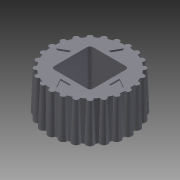
# Autodesk Inventor part: Shaft Lock Bar Insert
Saved by Autodesk Inventor 2013 (Build 170138000, 138)
## iProperties
Created: 2010-06-22
Part Number: Shaft Lock Bar Insert
Document SubType Name: Modeling
Designer: Phil
Density: 1 g/cm^3
Material: Generic
Author: Phil
Autodesk Inventor part; units mm, degrees
ref_plane "YZ Plane" through (0, 0, 0) normal (1, 0, 0) x (0, 1, 0)
ref_plane "XZ Plane" through (0, 0, 0) normal (0, 1, 0) x (-1, 0, 0)
ref_plane "XY Plane" through (0, 0, 0) normal (0, 0, 1) x (1, 0, 0)
sketch "Sketch1" plane through (0, 0, 0) normal (0, 0, 1) x (1, 0, 0)
  arc A0 (-3.0987, -0.2197) -> (-3.05, -0.5898) centre (0, 0) ccw projected
  arc A1 (-3.0987, 0.2197) -> (-3.0987, -0.2197) centre (-3.14, 0) ccw projected
  arc A2 (-3.05, 0.5898) -> (-3.0987, 0.2197) centre (0, 0) ccw projected
  arc A3 (-2.9362, 1.0142) -> (-3.05, 0.5898) centre (-3.033, 0.8127) ccw projected
  arc A4 (-2.7934, 1.3591) -> (-2.9362, 1.0142) centre (0, 0) ccw projected
  arc A5 (-2.5737, 1.7396) -> (-2.7934, 1.3591) centre (-2.7193, 1.57) ccw projected
  arc A6 (-2.3465, 2.0357) -> (-2.5737, 1.7396) centre (0, 0) ccw projected
  arc A7 (-2.0357, 2.3465) -> (-2.3465, 2.0357) centre (-2.2203, 2.2203) ccw projected
  arc A8 (-1.7396, 2.5737) -> (-2.0357, 2.3465) centre (0, 0) ccw projected
  arc A9 (-1.3591, 2.7934) -> (-1.7396, 2.5737) centre (-1.57, 2.7193) ccw projected
  arc A10 (-1.0142, 2.9362) -> (-1.3591, 2.7934) centre (0, 0) ccw projected
  arc A11 (-0.5898, 3.05) -> (-1.0142, 2.9362) centre (-0.8127, 3.033) ccw projected
  arc A12 (-0.2197, 3.0987) -> (-0.5898, 3.05) centre (0, 0) ccw projected
  arc A13 (0.2197, 3.0987) -> (-0.2197, 3.0987) centre (0, 3.14) ccw projected
  arc A14 (0.5892, 3.0501) -> (0.2197, 3.0987) centre (0, 0) ccw projected
  arc A15 (1.0148, 2.9361) -> (0.5892, 3.0501) centre (0.8119, 3.03) ccw projected
  arc A16 (1.3586, 2.7937) -> (1.0148, 2.9361) centre (0, 0) ccw projected
  arc A17 (1.7401, 2.5734) -> (1.3586, 2.7937) centre (1.5684, 2.7166) ccw projected
  arc A18 (2.0353, 2.3468) -> (1.7401, 2.5734) centre (0, 0) ccw projected
  arc A19 (2.3468, 2.0353) -> (2.0353, 2.3468) centre (2.2181, 2.2181) ccw projected
  arc A20 (2.5734, 1.7401) -> (2.3468, 2.0353) centre (0, 0) ccw projected
  arc A21 (2.7937, 1.3586) -> (2.5734, 1.7401) centre (2.7166, 1.5684) ccw projected
  arc A22 (2.9361, 1.0148) -> (2.7937, 1.3586) centre (0, 0) ccw projected
  arc A23 (3.0501, 0.5892) -> (2.9361, 1.0148) centre (3.03, 0.8119) ccw projected
  arc A24 (3.0987, 0.2203) -> (3.0501, 0.5892) centre (0, 0) ccw projected
  arc A25 (3.0987, -0.2203) -> (3.0987, 0.2203) centre (3.1369, 0) ccw projected
  arc A26 (3.05, -0.5898) -> (3.0987, -0.2203) centre (0, 0) ccw projected
  arc A27 (2.9362, -1.0142) -> (3.05, -0.5898) centre (3.033, -0.8127) ccw projected
  arc A28 (2.7934, -1.3591) -> (2.9362, -1.0142) centre (0, 0) ccw projected
  arc A29 (2.5737, -1.7396) -> (2.7934, -1.3591) centre (2.7193, -1.57) ccw projected
  arc A30 (2.3465, -2.0357) -> (2.5737, -1.7396) centre (0, 0) ccw projected
  arc A31 (2.0357, -2.3465) -> (2.3465, -2.0357) centre (2.2203, -2.2203) ccw projected
  arc A32 (1.7396, -2.5737) -> (2.0357, -2.3465) centre (0, 0) ccw projected
  arc A33 (1.3591, -2.7934) -> (1.7396, -2.5737) centre (1.57, -2.7193) ccw projected
  arc A34 (1.0142, -2.9362) -> (1.3591, -2.7934) centre (0, 0) ccw projected
  arc A35 (0.5898, -3.05) -> (1.0142, -2.9362) centre (0.8127, -3.033) ccw projected
  arc A36 (0.2197, -3.0987) -> (0.5898, -3.05) centre (0, 0) ccw projected
  arc A37 (-0.2197, -3.0987) -> (0.2197, -3.0987) centre (0, -3.14) ccw projected
  arc A38 (-0.5898, -3.05) -> (-0.2197, -3.0987) centre (0, 0) ccw projected
  arc A39 (-1.0142, -2.9362) -> (-0.5898, -3.05) centre (-0.8127, -3.033) ccw projected
  arc A40 (-1.3591, -2.7934) -> (-1.0142, -2.9362) centre (0, 0) ccw projected
  arc A41 (-1.7396, -2.5737) -> (-1.3591, -2.7934) centre (-1.57, -2.7193) ccw projected
  arc A42 (-2.0357, -2.3465) -> (-1.7396, -2.5737) centre (0, 0) ccw projected
  arc A43 (-2.3465, -2.0357) -> (-2.0357, -2.3465) centre (-2.2203, -2.2203) ccw projected
  arc A44 (-2.5737, -1.7396) -> (-2.3465, -2.0357) centre (0, 0) ccw projected
  arc A45 (-2.7934, -1.3591) -> (-2.5737, -1.7396) centre (-2.7193, -1.57) ccw projected
  arc A46 (-2.9362, -1.0142) -> (-2.7934, -1.3591) centre (0, 0) ccw projected
  arc A47 (-3.05, -0.5898) -> (-2.9362, -1.0142) centre (-3.033, -0.8127) ccw projected
  circle A48 centre (5.8886, 0) radius 1 projected
  line L0 (-5.4864, 0.8763) -> (-3.9624, 0) projected
  line L1 (-3.9624, 0) -> (-5.4864, -0.8763) projected
  line L2 (-5.4864, -0.8763) -> (-5.4864, 0.8763) projected
  circle A49 centre (-12.7, 0) radius 2.3114 projected
  circle A50 centre (12.7, 0) radius 2.3114 projected
  line L3 (3.7915, -5.0246) -> (16.487, -5.0246) projected
  line L4 (16.487, -5.0246) -> (17.7246, -3.787) projected
  line L5 (17.7246, -3.787) -> (17.7246, 3.787) projected
  line L6 (17.7246, 3.787) -> (16.487, 5.0246) projected
  line L7 (16.487, 5.0246) -> (3.7915, 5.0246) projected
  arc A51 (3.7915, 5.0246) -> (-3.7915, 5.0246) centre (0, 0) ccw projected
  line L8 (-3.7915, 5.0246) -> (-16.487, 5.0246) projected
  line L9 (-16.487, 5.0246) -> (-17.7246, 3.787) projected
  line L10 (-17.7246, 3.787) -> (-17.7246, -3.787) projected
  line L11 (-17.7246, -3.787) -> (-16.487, -5.0246) projected
  line L12 (-16.487, -5.0246) -> (-3.7915, -5.0246) projected
  arc A52 (-3.7915, -5.0246) -> (3.7915, -5.0246) centre (0, 0) ccw projected
  point P0 (0, 0)
extrude "Extrusion1" add sketch "Sketch1" against normal blind 3.175 draft 2 contours A1 A2 A3 A4 A5 A6 A7 A8 A9 A10 A11 A12 A13 A14 A15 A16 A17 A18 A19 A20 A21 A22 A23 A24 A25 A26 A27 A28 A29 A30 A31 A32 A33 A34 A35 A36 A37 A38 A39 A40 A41 A42 A43 A44 A45 A46 A47 A0
sketch "Sketch3" plane through (0, 0, -3.175) normal (0, 0, -1) x (-1, 0, 0)
  line L0 (-1.6125, -1.3625) -> (-1.6125, 1.3625)
  arc A0 (-1.3625, 1.6125) -> (-1.6125, 1.3625) centre (-1.3625, 1.3625) ccw
  line L1 (-1.3625, 1.6125) -> (1.3625, 1.6125)
  arc A1 (1.6125, 1.3625) -> (1.3625, 1.6125) centre (1.3625, 1.3625) ccw
  line L2 (1.6125, 1.3625) -> (1.6125, -1.3625)
  arc A2 (1.3625, -1.6125) -> (1.6125, -1.3625) centre (1.3625, -1.3625) ccw
  line L3 (1.3625, -1.6125) -> (-1.3625, -1.6125)
  arc A3 (-1.6125, -1.3625) -> (-1.3625, -1.6125) centre (-1.3625, -1.3625) ccw
  point P0 (0, 0)
  constraints: 8 end point, 8 point on circle, 4 centre point
extrude "Extrusion3" cut sketch "Sketch3" against normal through all
sketch "Sketch4" plane through (0, 0, 0) normal (0, 0, 1) x (1, 0, 0)
  line L0 (0, -2.8) -> (-0.45, -2)
  line L1 (-0.45, -2) -> (0.45, -2)
  line L2 (0.45, -2) -> (0, -2.8)
  line L3 (-0.45, 2) -> (0, 2.8)
  line L4 (0.45, 2) -> (-0.45, 2)
  line L5 (0, 2.8) -> (0.45, 2)
  line L6 (2.8, 0) -> (2, -0.45)
  line L7 (2, -0.45) -> (2, 0.45)
  line L8 (2.8, 0) -> (2, 0.45)
  line L9 (2, 0.45) -> (2.8, 0)
  line L10 (-2.8, 0) -> (-2, 0.45)
  line L11 (-2, -0.45) -> (-2.8, 0)
  line L12 (-2, 0.45) -> (-2, -0.45)
  line L13 (0, -2.8) -> (-0.45, -2)
  line L14 (-0.45, -2) -> (0.45, -2)
  line L15 (0.45, -2) -> (0, -2.8)
  line L16 (2.8, 0) -> (2, -0.45)
  line L17 (2, -0.45) -> (2, 0.45)
  line L18 (2.8, 0) -> (2, 0.45)
  line L19 (2, 0.45) -> (2.8, 0)
  point P0 (0, 0)
  point P1 (0, 0)
  point P2 (0, 0)
  point P3 (0, 0)
  point P4 (0, 0)
  point P5 (0, 0)
  point P6 (0, 0)
  point P7 (0, 0)
  point P8 (0, 0)
  point P9 (0, 0)
  point P10 (0, 0)
  point P11 (0, 0)
  point P12 (0, 0)
  point P13 (0, 0)
  point P14 (0, 0)
  point P15 (0, 0)
  point P16 (0, 0)
  point P17 (0, 0)
  point P18 (0, 0)
  point P19 (0, 0)
  point P20 (0, 0)
  point P21 (0, 0)
  point P22 (0, 0)
  point P23 (0, 0)
  point P24 (0, 0)
  point P25 (0, 0)
  point P26 (0, 0)
  point P27 (0, 0)
  point P28 (0, 0)
  point P29 (0, 0)
  point P30 (0, 0)
  point P31 (0, 0)
  point P32 (0, 0)
  point P33 (0, 0)
  point P34 (0, 0)
  point P35 (0, 0)
  point P36 (0, 0)
  point P37 (0, 0)
  point P38 (0, 0)
  point P39 (0, 0)
  point P40 (0, 0)
  point P41 (0, 0)
  point P42 (0, 0)
  point P43 (0, 0)
  constraints: 40 end point
extrude "Extrusion4" cut sketch "Sketch4" against normal blind 0.127
sketch "Sketch5" plane through (0, 0, 0) normal (0, 0, 1) x (1, 0, 0)
  line L0 (-1.6125, -1.3625) -> (-1.6125, 1.3625) projected
  line L1 (-1.3625, 1.6125) -> (1.3625, 1.6125) projected
  line L2 (1.6125, 1.3625) -> (1.6125, -1.3625) projected
  line L3 (1.3625, -1.6125) -> (-1.3625, -1.6125) projected
  arc A0 (-3.05, 0.5898) -> (-3.0987, 0.2197) centre (0, 0) ccw projected
  circle A1 centre (0, 0) radius 1.6125
  constraints: 4 tangent, 1 centre point, 1 coincident
surface extrude "ExtrusionSrf1" sketch "Sketch5" against normal up to surface (3.175 mm away) shown no curves A1
body "Solid1"
body "Srf1"
